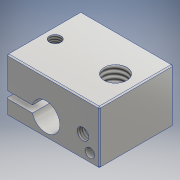
# Autodesk Inventor part: Heat Block
Saved by Autodesk Inventor 2016 (Build 200138000, 138)
## iProperties
Created: 2016-03-26
Part Number: Heat Block
Material: Aluminum 6061
Document SubType Name: Modeling
Designer: Scott
Mass: 7.52447 g
Surface Area: 20.5034 cm^2
Volume: 2.78684 cm^3
Density: 2.7 g/cm^3
Appearance: Aluminum - Flat
Author: Scott
Autodesk Inventor part; units mm, degrees
note: some values were not read from the file. Chosen so that the rebuilt part matches the saved one: direction of "Hole5"; direction of "Hole6".
ref_plane "YZ Plane" through (0, 0, 0) normal (1, 0, 0) x (0, 1, 0)
ref_plane "XZ Plane" through (0, 0, 0) normal (0, 1, 0) x (-1, 0, 0)
ref_plane "XY Plane" through (0, 0, 0) normal (0, 0, 1) x (1, 0, 0)
sketch "Sketch1" plane through (0, 0, 0) normal (0, 0, 1) x (1, 0, 0)
  line L0 (0, 0) -> (20, 0)
  line L1 (20, 0) -> (20, 16)
  line L2 (20, 16) -> (0, 16)
  line L3 (0, 16) -> (0, 0)
  dimension "d0" = 20
  dimension "d1" = 16
  constraints: 8 end point, 2 parallel, 1 horizontal, 1 perpendicular
  measures "d0" distance of L0.start L0.end
  measures "d1" distance of L0.end L1.end
extrude "Extrusion1" add sketch "Sketch1" along normal blind 11.5
sketch "Sketch2" plane through (0, 0, 11.5) normal (0, 0, 1) x (1, 0, 0)
  line L0 (20, 0) -> (20, 16) projected
  line L1 (0, 0) -> (20, 0) projected
  point P0 (15.5, 8)
  dimension "d4" = 4.5
  dimension "d5" = 8
  measures "d4" distance from line of L0 point (15.5, 8)
  measures "d5" distance from line of point (15.5, 8) L1
hole "Hole1" at (15.5, 8, 11.5) direction (0, 0, -1) diameter 4.917 end through all thread size "M6x1" class "6H" standard "ISO Metric profile"
sketch "Sketch3" plane through (0, 0, 0) normal (0, -1, 0) x (1, 0, 0)
  arc A0 (5.5953, 3.25) -> (5.5953, 4.75) centre (8.5, 4) ccw
  line L0 (0, 0) -> (20, 0) projected
  line L1 (20, 0) -> (20, 11.5) projected
  line L2 (0, 0) -> (0, 11.5) projected
  line L3 (0, 4.75) -> (5.5953, 4.75)
  line L4 (0, 3.25) -> (5.5953, 3.25)
  dimension "d13" = 4
  dimension "d14" = 11.5
  dimension "d15" = 3
  dimension "d16" = 0.75
  dimension "d17" = 0.75
  constraints: 4 end point, 2 point on circle, 2 point on line, 1 centre point, 1 horizontal, 1 perpendicular
  measures "d13" distance from line of L0 A0.centre
  measures "d14" distance from line of A0.centre L1
  measures "d15" radius of A0
  measures "d16" distance from line of L3 A0.centre
  measures "d17" distance from line of L4 A0.centre
extrude "Extrusion2" cut sketch "Sketch3" against normal through all
sketch "Sketch4" plane through (0, 0, 0) normal (0, -1, 0) x (1, 0, 0)
  line L0 (0, 0) -> (20, 0) projected
  line L1 (20, 0) -> (20, 11.5) projected
  point P0 (16.5, 4.8)
  point P1 (18, 2)
  dimension "d20" = 4.8
  dimension "d21" = 3.5
  dimension "d22" = 2
  dimension "d23" = 2
  measures "d20" distance from line of point (16.5, 4.8) L0
  measures "d21" distance from line of point (16.5, 4.8) L1
  measures "d22" distance from line of L1 point (18, 2)
  measures "d23" distance from line of L0 point (18, 2)
hole "Hole2" at (16.5, 0, 4.8) direction (0, 1, 0) diameter 2.459 depth 3.5 tip angle 118 thread size "M3x0.5" class "6H" standard "ISO Metric profile"
hole "Hole3" at (18, 0, 2) direction (0, 1, 0) diameter 1.5 depth 4.5 tip angle 118
hole "Hole4" at (18, 0, 2) direction (0, 1, 0) diameter 2 depth 2 tip angle 118
sketch "Sketch5" plane through (0, 0, 11.5) normal (0, 0, 1) x (1, 0, 0)
  line L0 (0, 0) -> (20, 0) projected
  line L1 (20, 0) -> (20, 16) projected
  point P0 (2.5, 8)
  dimension "d45" = 8
  dimension "d46" = 17.5
  measures "d45" distance from line of point (2.5, 8) L0
  measures "d46" distance from line of L1 point (2.5, 8)
hole "Hole5" at (2.5, 8, 11.5) direction (0, 0, -1) diameter 2.459 end up to surface thread size "M3x0.5" class "6H" standard "ISO Metric profile"
sketch "Sketch6" plane through (0, 0, 0) normal (0, 0, -1) x (-1, 0, 0)
  circle A0 centre (-2.5, 8) radius 1.2295 projected
  point P0 (0, 0)
hole "Hole6" at (2.5, 8, 0) direction (0, 0, 1) diameter 3 end up to surface
chamfer "Chamfer1" distance 0.25 angle 45 14 edges at (0, 8, 11.5) (0, 16, 8.125) (0, 16, 1.625) (0, 8, 0) (0, 0, 1.625) (0, 0, 8.125) (10, 0, 11.5) (10, 0, 0) (20, 0, 5.75) (20, 8, 11.5) (10, 16, 11.5) (20, 8, 0) (20, 16, 5.75) (10, 16, 0)
equation "\"d17\" = d16"
body "Solid1"
